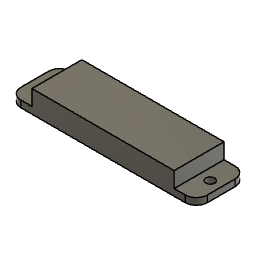
cross_support (Autodesk Fusion 360 design; units mm, degrees)
Autodesk Fusion 360 part; units mm, degrees
sketch "Sketch1" plane through (0, 0, 0) normal (0, 1, 0) x (1, 0, 0)
  line L0 (0, 0) -> (64.11, 0)
  line L1 (64.11, 0) -> (64.11, -22.5)
  line L2 (64.11, -22.5) -> (0, -22.5)
  line L3 (0, -22.5) -> (0, 0)
  line L4 (0, -11.25) -> (-5, -11.25) construction
  circle A0 centre (-5, -11.25) radius 2
  line L5 (0, -14.9977) -> (0, 0)
  line L6 (64.11, -11.25) -> (69.11, -11.25) construction
  circle A1 centre (69.11, -11.25) radius 2
  line L7 (64.11, -15) -> (64.11, 0)
  line L8 (64.11, 0) -> (69.11, 0)
  line L9 (74.11, -5) -> (74.11, -17.5)
  line L10 (69.11, -22.5) -> (64.11, -22.5)
  line L11 (64.11, -22.5) -> (64.11, 0)
  arc A2 (74.11, -5) -> (69.11, 0) centre (69.11, -5) ccw
  arc A3 (69.11, -22.5) -> (74.11, -17.5) centre (69.11, -17.5) ccw
  line L12 (0, 0) -> (-5, 0)
  line L13 (-10, -5) -> (-10, -17.5)
  line L14 (-5, -22.5) -> (0, -22.5)
  line L15 (0, -22.5) -> (0, 0)
  arc A4 (-5, 0) -> (-10, -5) centre (-5, -5) ccw
  arc A5 (-10, -17.5) -> (-5, -22.5) centre (-5, -17.5) ccw
  point P0 (74.11, 0)
  point P1 (-10, 0)
  dimension "d1" = 64.11
  dimension "d2" = 22.5
  dimension "d3" = 5
  dimension "d4" = 4
  dimension "d7" = 5
  dimension "d8" = 4
  dimension "d15" = 10
  dimension "d16" = 5
  dimension "d17" = 10
  dimension "d18" = 5
  constraint horizontal L0
  constraint vertical L1
  constraint horizontal L2
  constraint vertical L3
  constraint coincident L0.start L3.end
  constraint midpoint L3 L4.start
  constraint perpendicular L3 L4
  constraint coincident L4.end A0.centre
  constraint vertical L5
  constraint midpoint L1 L6.start
  constraint perpendicular L1 L6
  constraint coincident L6.end A1.centre
  constraint vertical L7
  constraint horizontal L8
  constraint vertical L9
  constraint horizontal L10
  constraint vertical L11
  constraint coincident P0 L8
  constraint coincident P0 L9
  constraint tangent L8 A2
  constraint tangent L9 A2
  constraint tangent L10 A3
  constraint tangent L9 A3
  constraint equal A2 A3
  constraint horizontal L12
  constraint vertical L13
  constraint horizontal L14
  constraint vertical L15
  constraint coincident P1 L12
  constraint coincident P1 L13
  constraint tangent L12 A4
  constraint tangent L13 A4
  constraint tangent L14 A5
  constraint tangent L13 A5
  constraint equal A4 A5
  measures "d1" distance of L0.start L0.end
  measures "d2" distance of L0.start L2.end
  measures "d3" distance of L4.start L4.end
  measures "d4" diameter of A0
  measures "d7" distance of L6.start L6.end
  measures "d8" diameter of A1
  measures "d15" distance of L0.end P0
  measures "d16" radius of A2
  measures "d17" distance of L0.start P1
  measures "d18" radius of A4
extrude "Extrude1" add sketch "Sketch1" along normal blind 10 contours L0 L1 L2 L3 L5 L7 L11 L15
extrude "Extrude2" add sketch "Sketch1" along normal blind 3 contours L3 L5 L12 L13 L14 L15 A4 A5 | L1 L7 L8 L9 L10 L11 A2 A3
named bodies: "cross_support"
